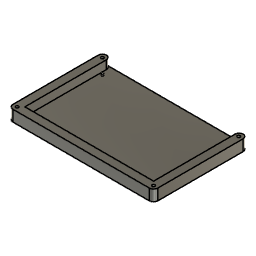
FloppySquare Base (Autodesk Fusion 360 design; units mm, degrees)
part number: 2025-07-31-18-04-11-539
part number: 2025-07-31-18-07-05-915
Autodesk Fusion 360 part; units mm, degrees
sketch "Sketch1" plane through (0, 0, 0) normal (0, 0, 1) x (1, 0, 0) in component "FloppySquare Base (1)"
  line L0 (0, 0) -> (151, 0)
  line L1 (151, 0) -> (151, 100.5)
  line L2 (151, 100.5) -> (0, 100.5)
  line L3 (0, 100.5) -> (0, 0)
  line L4 (-9.5, 0) -> (160.5, 0)
  line L5 (160.5, 0) -> (160.5, 110)
  line L6 (160.5, 110) -> (-9.5, 110)
  line L7 (-9.5, 110) -> (-9.5, 0)
  circle A0 centre (-4.5, 105) radius 1.7
  circle A1 centre (-4.5, 5) radius 1.7
  circle A2 centre (155.5, 5) radius 1.7
  circle A3 centre (155.5, 105) radius 1.7
  circle A4 centre (-4.5, 105) radius 3
  circle A5 centre (-4.5, 5) radius 3
  circle A6 centre (155.5, 5) radius 3
  circle A7 centre (155.5, 105) radius 3
  circle A8 centre (147.5, 13) radius 1.25
  circle A9 centre (147.5, 97) radius 1.25
  circle A10 centre (3.5, 97) radius 1.25
  circle A11 centre (3.5, 13.5) radius 1.25
  dimension "d1" = 151
  dimension "d2" = 100.5
  dimension "d3" = 110
  dimension "d4" = 9.5
  dimension "d5" = 9.5
  dimension "d6" = 3.4
  dimension "d7" = 3.4
  dimension "d8" = 3.4
  dimension "d9" = 3.4
  dimension "d10" = 5
  dimension "d11" = 5
  dimension "d12" = 5
  dimension "d13" = 5
  dimension "d14" = 5
  dimension "d15" = 5
  dimension "d16" = 5
  dimension "d17" = 5
  dimension "d18" = 6
  dimension "d19" = 6
  dimension "d20" = 6
  dimension "d21" = 6
  dimension "d31" = 2.5
  dimension "d32" = 13
  dimension "d33" = 3.5
  dimension "d34" = 2.5
  dimension "d35" = 3.5
  dimension "d36" = 3.5
  dimension "d37" = 2.5
  dimension "d38" = 3.5
  dimension "d39" = 3.5
  dimension "d40" = 2.5
  dimension "d41" = 13.5
  dimension "d42" = 3.5
  constraint horizontal L0
  constraint vertical L1
  constraint horizontal L2
  constraint vertical L3
  constraint coincident L0.start L3.end
  constraint horizontal L4
  constraint vertical L5
  constraint horizontal L6
  constraint vertical L7
  constraint concentric A0 A4
  constraint concentric A1 A5
  constraint concentric A2 A6
  constraint concentric A3 A7
  measures "d1" distance of L0.start L0.end
  measures "d2" distance of L0.start L2.end
  measures "d3" distance of L4.start L6.end
  measures "d4" distance of L2 L6
  measures "d5" distance of L3 L7
  measures "d6" diameter of A0
  measures "d7" diameter of A1
  measures "d8" diameter of A2
  measures "d9" diameter of A3
  measures "d10" distance of L6 A0.centre
  measures "d11" distance of L7 A0.centre
  measures "d12" distance of L4 A1.centre
  measures "d13" distance of L7 A1.centre
  measures "d14" distance of L4 A2.centre
  measures "d15" distance of L5 A2.centre
  measures "d16" distance of L6 A3.centre
  measures "d17" distance of L5 A3.centre
  measures "d18" diameter of A4
  measures "d19" diameter of A5
  measures "d20" diameter of A6
  measures "d21" diameter of A7
  measures "d31" diameter of A8
  measures "d32" distance of L0 A8.centre
  measures "d33" distance of L1 A8.centre
  measures "d34" diameter of A9
  measures "d35" distance of L2 A9.centre
  measures "d36" distance of L1 A9.centre
  measures "d37" diameter of A10
  measures "d38" distance of L2 A10.centre
  measures "d39" distance of L3 A10.centre
  measures "d40" diameter of A11
  measures "d41" distance of L0 A11.centre
  measures "d42" distance of L3 A11.centre
extrude "Extrude1" add sketch "Sketch1" along normal blind 9.9 from surface at 3.1 contours A4 | A5 | A6 | A7 makes body 1 at (157.7981, 6.9284, 9.7) makes body 2 at (152.7356, 103.8347, 9.7) makes body 3 at (-1.5037, 4.8505, 9.7) makes body 4 at (-7.2644, 103.8347, 9.7) in component "FloppySquare Base (1)"
extrude "Extrude2" add sketch "Sketch1" along normal blind 13 contours L1 L2 L3 L4 L5 L6 L7 bodies 1 2 3 4 in component "FloppySquare Base (1)"
extrude "Extrude3" add sketch "Sketch1" along normal blind 3 contours L0 L1 L2 L3 L4 | A8 | A9 | A10 | A11 bodies 1 in component "FloppySquare Base (1)"
fillet "Fillet1" radius 5 4 edges at (160.5, 110, 6.5) (160.5, 0, 6.5) (-9.5, 0, 6.5) (-9.5, 110, 6.5) on bodies 1 in component "FloppySquare Base (1)"
extrude "Extrude4" add sketch "Sketch1" along normal blind 6 contours A8 | A9 | A10 | A11 bodies 1 in component "FloppySquare Base (1)"
fillet "Fillet2" radius 1 4 edges at (146.3346, 96.548, 6) (146.3346, 12.548, 6) (2.3346, 13.048, 6) (2.3346, 96.548, 6) on bodies 1 in component "FloppySquare Base (1)"
fillet "Fillet3" radius 5 2 edges at (0, 0, 8) (151, 0, 8) on bodies 1 in component "FloppySquare Base (1)"
move_body "Move1" bodies 1 to x (-1, 0, 0) y (0, -1, 0) z (0, 0, 1) at (-19, 0, 0) in component "FloppySquare Base (1)"
component "FloppySquare Base (1)" placed x (1, 0, 0) y (0, 1, 0) z (0, 0, 1) at (0, 0, 0)
